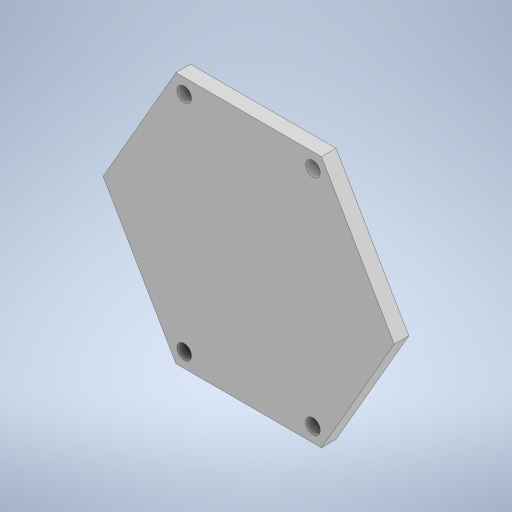
# Autodesk Inventor part: ArmControlBoard
Saved by Autodesk Inventor 2023 (Build 270158000, 158)
## iProperties
Created: 2023-11-22
Part Number: ArmControlBoard
Material: Generic
Document SubType Name: Modeling
Designer: LattePanda
Density: 1 g/cm^3
Appearance: Default
Author: LattePanda
Autodesk Inventor part; units mm, degrees
ref_plane "YZ Plane" through (0, 0, 0) normal (1, 0, 0) x (0, 1, 0)
ref_plane "XZ Plane" through (0, 0, 0) normal (0, 1, 0) x (-1, 0, 0)
ref_plane "XY Plane" through (0, 0, 0) normal (0, 0, 1) x (1, 0, 0)
sketch "Sketch1" plane through (0, 0, 0) normal (0, 0, 1) x (1, 0, 0)
  line L0 (-29.9999, 0.0001) -> (-15, -25.9807)
  line L1 (15, -25.9808) -> (30, 0)
  line L2 (-15, -25.9807) -> (15, -25.9808)
  line L3 (30, 0) -> (15, 25.9808)
  line L4 (15, 25.9808) -> (-15, 25.9808)
  line L5 (-15, 25.9808) -> (-30, 0)
  line L6 (0, 25.9808) -> (0, -25.9808) construction
  line L7 (-30, 0) -> (30, 0) construction
  line L8 (-24.8039, 3) -> (-13.268, 22.9808) construction
  line L9 (-13.268, 22.9808) -> (13.2679, 22.9808) construction
  line L10 (13.2679, 22.9808) -> (24.8038, 3) construction
  line L11 (24.8038, 3) -> (-24.8039, 3) construction
  circle A0 centre (-13.268, 22.9808) radius 1.5
  circle A1 centre (13.2679, 22.9808) radius 1.5
  circle A2 centre (-24.8039, 0) radius 1.5 construction
  line L12 (-24.8039, 3) -> (-26.5359, 0) construction
  circle A3 centre (24.8039, 0.0001) radius 1.5 construction
  circle A4 centre (-13.268, -22.9808) radius 1.5
  circle A5 centre (13.2679, -22.9808) radius 1.5
  point P0 (0, 0)
  point P1 (0, 0)
  point P2 (-30, 0.0001)
  dimension "d1" = 30
  dimension "d6" = 120
  dimension "d7" = 120
  dimension "d8" = 120
  dimension "d9" = 120
  dimension "d10" = 120
  dimension "d13" = 3
  dimension "d14" = 3
  dimension "d15" = 3
  constraints: 26 end point, 6 centre point, 5 equal length, 3 coincident, 3 midpoint, 3 symmetric about line, 2 point on line, 1 collinear, 1 equal radius, 1 horizontal, 1 tangent, 6 other
  measures "d1" distance of L3.end L4.end
  measures "d6" angle of L4 L5
  measures "d7" angle of L3 L4
  measures "d8" angle of L0 L5
  measures "d9" angle of L1 L3
  measures "d10" angle of L2 L0
  measures "d13" distance between parallel lines of L5 L8
  measures "d14" diameter of A0
  measures "d15" diameter of A1
extrude "Extrusion1" add sketch "Sketch1" along normal blind 3
equation "\"d7\" = d6"
equation "\"d8\" = d6"
equation "\"d9\" = d6"
equation "\"d10\" = d6"
body "Solid1"
